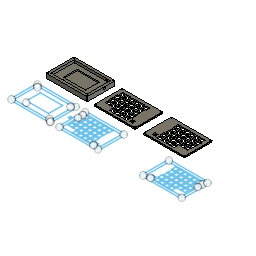
KEYBOARD_SPLIT (Autodesk Fusion 360 design; units mm, degrees)
part number: 2026-05-08-19-29-42-942
Autodesk Fusion 360 part; units mm, degrees
sketch "Sketch1" plane through (0, 0, 0) normal (0, 1, 0) x (1, 0, 0)
  line L0 (45, 19.9678) -> (192.4, 19.9678)
  line L1 (192.4, 19.9678) -> (192.4, -74.4322)
  line L2 (192.4, -74.4322) -> (45, -74.4322)
  line L3 (45, -74.4322) -> (45, 19.9678)
  line L4 (35, -84.4322) -> (35, 29.9678)
  line L5 (35, 29.9678) -> (202.4, 29.9678)
  line L6 (202.4, 29.9678) -> (202.4, -84.4322)
  line L7 (202.4, -84.4322) -> (35, -84.4322)
  line L8 (75, 2.7892) -> (165, 2.7892)
  line L9 (165, 2.7892) -> (165, -54.0461)
  line L10 (165, -54.0461) -> (75, -54.0461)
  line L11 (75, -54.0461) -> (75, 2.7892)
  line L12 (38, 27) -> (38, 23)
  line L13 (42, 23) -> (42, 27)
  line L14 (42, 27) -> (38, 27)
  line L15 (38, 23) -> (42, 23)
  line L16 (38, -78) -> (38, -82)
  line L17 (38, -82) -> (42, -82)
  line L18 (42, -82) -> (42, -78)
  line L19 (42, -78) -> (38, -78)
  line L20 (195.5084, -78) -> (195.5084, -82)
  line L21 (195.5084, -82) -> (199.5084, -82)
  line L22 (199.5084, -82) -> (199.5084, -78)
  line L23 (199.5084, -78) -> (195.5084, -78)
  line L24 (195.5084, 23.0262) -> (199.5084, 23.0262)
  line L25 (199.5084, 23.0262) -> (199.5084, 27.0262)
  line L26 (195.5084, 23.0262) -> (195.5084, 27.0262)
  line L27 (195.5084, 27.0262) -> (199.5084, 27.0262)
  point P0 (40, 25)
  point P1 (197.5, 25)
  point P2 (197.5, -80)
  point P3 (40, -80)
  point P4 (186.4, 13.9678)
  point P5 (186.4, -71.7)
  point P6 (80.7091, -61.1944)
  point P7 (49.5091, 16.0056)
  dimension "d1" = 147.4
  dimension "d2" = 94.4
  dimension "d3" = 147.4
  dimension "d6" = -10
  dimension "d24" = 4
  dimension "d25" = 4
  dimension "d26" = 4
  constraint horizontal L0
  constraint perpendicular L0 L1
  constraint perpendicular L1 L2
  constraint horizontal L8
  constraint vertical L9
  constraint horizontal L10
  constraint vertical L11
  constraint vertical L12
  constraint parallel L12 L13
  constraint perpendicular L13 L14
  constraint perpendicular L13 L15
  constraint perpendicular L15 L16
  constraint perpendicular L16 L17
  constraint perpendicular L17 L18
  constraint perpendicular L16 L19
  constraint vertical L20
  constraint perpendicular L20 L21
  constraint perpendicular L21 L22
  constraint perpendicular L20 L23
  constraint perpendicular L20 L24
  constraint perpendicular L24 L25
  constraint perpendicular L24 L26
  measures "d1" distance of L0.start L0.end
  measures "d2" distance of L0.end L1.end
  measures "d3" distance of L1.end L2.end
  measures "d24" distance of L24.start L24.end
  measures "d25" distance of L24.end L25.end
  measures "d26" distance of L24.start L26.end
extrude "Extrude1" add sketch "Sketch1" along normal blind 3 contours L0 L1 L2 L3 | L4 L5 L6 L7 | L8 L9 L10 L11 | L12 L13 L14 L15 | L16 L17 L18 L19 | L20 L21 L22 L23 | L24 L25 L26 L27 makes body 1
extrude "Extrude2" add sketch "Sketch1" along normal blind 8 separate body contours L0 L1 L2 L3 | L4 L5 L6 L7 | L12 L13 L14 L15 | L16 L17 L18 L19 | L20 L21 L22 L23 | L24 L25 L26 L27 makes body 2
extrude "Extrude3" add sketch "Sketch1" along normal blind 18 separate body contours L4 L5 L6 L7 | L12 L13 L14 L15 | L16 L17 L18 L19 | L20 L21 L22 L23 | L24 L25 L26 L27 makes body 3
combine "Combine1" operation add target body 1 tool bodies 2 3
hole "Hole1" at (49.5091, 0, -16.0056) at (80.7091, 0, 61.1944) at (186.4, 0, 71.7) at (186.4, 0, -13.9678) direction (0, 1, 0) diameter 2.4 end through all bodies 1
hole "Hole2" at (40, 0, -25) at (40, 0, 80) at (197.5, 0, -25) at (197.5, 0, 80) direction (0, 1, 0) diameter 2.4 end through all bodies 1
extrude "Extrude4" add sketch "Sketch1" along normal blind 3 separate body contours L12 L13 L14 L15 | L16 L17 L18 L19 | L20 L21 L22 L23 | L24 L25 L26 L27 makes body 4 at (196.8417, 0, 79.3333) makes body 5 at (39.3333, 0, 79.3333) makes body 6 at (196.8417, 0, -25.6929) makes body 7 at (39.3333, 0, -25.6667)
combine "Combine2" operation cut target body 1 tool bodies 4 5 6 7
sketch "Sketch2" plane through (0, 0, 0) normal (0, 1, 0) x (1, 0, 0)
  line L0 (220, 15) -> (229.1, 15)
  line L1 (229.1, 15) -> (229.1, -5)
  line L2 (229.1, -5) -> (220, -5)
  line L3 (220, -5) -> (220, 15)
  dimension "d29" = 9.1
  constraint horizontal L0
  constraint vertical L1
  constraint horizontal L2
  constraint vertical L3
  measures "d29" distance of L0.start L0.end
extrude "Extrude5" add sketch "Sketch2" along normal blind 3.4 separate body makes body 8
fillet "Fillet1" radius 0.5 4 edges at (229.1, 3.4, -5) (220, 3.4, -5) (229.1, 0, -5) (220, 0, -5) on bodies 8
move_body "Move1" bodies 8 to x (1, 0, 0) y (0, 1, 0) z (0, 0, 1) at (-48, 7.5, -20)
move_body "Move2" bodies 8 to x (1, 0, 0) y (0, 1, 0) z (0, 0, 1) at (0, 2, 0)
combine "Combine3" operation cut target body 1 tool bodies 8
fillet "Fillet2" radius 2 4 edges at (202.4, 9, -29.9678) (35, 9, -29.9678) (35, 9, 84.4322) (202.4, 9, 84.4322) on bodies 1
move_body "Move3" bodies 1 to x (1, 0, 0) y (0, 1, 0) z (0, 0, 1) at (0, 0, -150)
sketch "Sketch3" plane through (0, 0, 0) normal (0, 1, 0) x (1, 0, 0)
  line L0 (220, -20) -> (225, -20)
  line L1 (225, -20) -> (225, -28)
  line L2 (225, -28) -> (220, -28)
  line L3 (220, -28) -> (220, -20)
  dimension "d36" = 5
  dimension "d37" = 8
  constraint horizontal L0
  constraint vertical L1
  constraint horizontal L2
  constraint vertical L3
  measures "d36" distance of L0.start L0.end
  measures "d37" distance of L0.start L2.end
extrude "Extrude7" add sketch "Sketch3" along normal blind 20 separate body makes body 9
move_body "Move4" bodies 9 to x (0, 1, 0) y (-1, 0, 0) z (0, 0, 1) at (220, -220, 0)
move_body "Move5" bodies 9 to x (1, 0, 0) y (0, 1, 0) z (0, 0, 1) at (15, 10, -150)
move_body "Move6" bodies 9 to x (1, 0, 0) y (0, 1, 0) z (0, 0, 1) at (-27, -2, -12)
move_body "Move7" bodies 9 to x (1, 0, 0) y (0, 1, 0) z (0, 0, 1) at (0, 1, 0)
combine "Combine4" operation cut target body 1 tool bodies 9
sketch "Sketch4Sketch4" plane through (0, 0, 0) normal (0, 1, 0) x (1, 0, 0)
  line L0 (240, 20) -> (387.4, 20)
  line L1 (240, 20) -> (240, -74.4)
  line L2 (387.4, 20) -> (387.4, -74.4)
  line L3 (240, -74.4) -> (387.4, -74.4)
  line L4 (397.4, 30) -> (397.4, -84.4)
  line L5 (230, -84.4) -> (397.4, -84.4)
  line L6 (230, 30) -> (230, -84.4)
  line L7 (230, 30) -> (397.4, 30)
  line L8 (240, 20) -> (240, 9.6)
  line L9 (246.65, 9.6) -> (246.65, 16.65)
  line L10 (246.65, 16.65) -> (260.75, 16.65)
  line L11 (260.75, 16.65) -> (260.75, 2.55)
  line L12 (260.75, 2.55) -> (246.65, 2.55)
  line L13 (246.65, 2.55) -> (246.65, 9.6)
  line L14 (265.7, 16.65) -> (279.8, 16.65)
  line L15 (279.8, 16.65) -> (279.8, 2.55)
  line L16 (279.8, 2.55) -> (265.7, 2.55)
  line L17 (265.7, 2.55) -> (265.7, 16.65)
  line L18 (284.7517, 16.65) -> (298.8517, 16.65)
  line L19 (298.8517, 16.65) -> (298.8517, 2.55)
  line L20 (298.8517, 2.55) -> (284.7517, 2.55)
  line L21 (284.7517, 2.55) -> (284.7517, 16.65)
  line L22 (303.8299, 16.65) -> (317.9299, 16.65)
  line L23 (317.9299, 16.65) -> (317.9299, 2.65)
  line L24 (317.9299, 2.65) -> (303.8299, 2.65)
  line L25 (303.8299, 2.65) -> (303.8299, 16.65)
  line L26 (322.8799, 2.65) -> (322.8799, 16.65)
  line L27 (322.8799, 16.65) -> (336.9799, 16.65)
  line L28 (336.9799, 2.65) -> (322.8799, 2.65)
  line L29 (336.9799, 16.65) -> (336.9799, 2.65)
  line L30 (341.9299, 2.65) -> (341.9299, 16.65)
  line L31 (341.9299, 16.65) -> (356.0299, 16.65)
  line L32 (356.0299, 2.65) -> (341.9299, 2.65)
  line L33 (356.0299, 16.65) -> (356.0299, 2.65)
  line L34 (240, 20) -> (240, -9.43)
  line L35 (244.12, -9.43) -> (244.12, -2.38)
  line L36 (244.12, -2.38) -> (258.22, -2.38)
  line L37 (258.22, -2.38) -> (258.22, -16.48)
  line L38 (258.22, -16.48) -> (244.12, -16.48)
  line L39 (244.12, -16.48) -> (244.12, -9.43)
  line L40 (263.0302, -2.38) -> (277.1302, -2.38)
  line L41 (277.1302, -2.38) -> (277.1302, -16.48)
  line L42 (277.1302, -16.48) -> (263.0302, -16.48)
  line L43 (263.0302, -16.48) -> (263.0302, -2.38)
  line L44 (282.0802, -16.48) -> (282.0802, -2.38)
  line L45 (282.0802, -2.38) -> (296.1802, -2.38)
  line L46 (296.1802, -2.38) -> (296.1802, -16.48)
  line L47 (296.1802, -16.48) -> (282.0802, -16.48)
  line L48 (301.1302, -16.48) -> (301.1302, -2.38)
  line L49 (315.2302, -16.48) -> (301.1302, -16.48)
  line L50 (315.2302, -2.38) -> (315.2302, -16.48)
  line L51 (301.1302, -2.38) -> (315.2302, -2.38)
  line L52 (320.1802, -16.48) -> (320.1802, -2.38)
  line L53 (320.1802, -2.38) -> (334.2802, -2.38)
  line L54 (334.2802, -16.48) -> (320.1802, -16.48)
  line L55 (334.2802, -2.38) -> (334.2802, -16.48)
  line L56 (339.2302, -16.48) -> (339.2302, -2.38)
  line L57 (353.3302, -16.48) -> (339.2302, -16.48)
  line L58 (353.3302, -2.38) -> (353.3302, -16.48)
  line L59 (339.2302, -2.38) -> (353.3302, -2.38)
  line L60 (244.12, -21.43) -> (258.22, -21.43)
  line L61 (244.12, -28.48) -> (244.12, -21.43)
  line L62 (244.12, -35.53) -> (244.12, -28.48)
  line L63 (258.22, -21.43) -> (258.22, -35.53)
  line L64 (277.1302, -21.43) -> (277.1302, -35.53)
  line L65 (258.22, -35.53) -> (244.12, -35.53)
  line L66 (263.0302, -35.53) -> (263.0302, -21.43)
  line L67 (263.0302, -21.43) -> (277.1302, -21.43)
  line L68 (282.0802, -35.53) -> (282.0802, -21.43)
  line L69 (277.1302, -35.53) -> (263.0302, -35.53)
  line L70 (339.2302, -35.53) -> (339.2302, -21.43)
  line L71 (301.1302, -21.43) -> (315.2302, -21.43)
  line L72 (315.2302, -21.43) -> (315.2302, -35.53)
  line L73 (353.3302, -21.43) -> (353.3302, -35.53)
  line L74 (315.2302, -35.53) -> (301.1302, -35.53)
  line L75 (339.2302, -21.43) -> (353.3302, -21.43)
  line L76 (320.1802, -35.53) -> (320.1802, -21.43)
  line L77 (334.2802, -21.43) -> (334.2802, -35.53)
  line L78 (334.2802, -35.53) -> (320.1802, -35.53)
  line L79 (353.3302, -35.53) -> (339.2302, -35.53)
  line L80 (320.1802, -21.43) -> (334.2802, -21.43)
  line L81 (301.1302, -35.53) -> (301.1302, -21.43)
  line L82 (296.1802, -21.43) -> (296.1802, -35.53)
  line L83 (296.1802, -35.53) -> (282.0802, -35.53)
  line L84 (282.0802, -21.43) -> (296.1802, -21.43)
  line L85 (246.65, -54.6) -> (246.65, -47.55)
  line L86 (265.7, -54.6) -> (265.7, -40.5)
  line L87 (265.7, -40.5) -> (279.8, -40.5)
  line L88 (260.75, -40.5) -> (260.75, -54.6)
  line L89 (246.65, -40.5) -> (260.75, -40.5)
  line L90 (260.75, -54.6) -> (246.65, -54.6)
  line L91 (279.8, -54.6) -> (265.7, -54.6)
  line L92 (284.7517, -54.6) -> (284.7517, -40.5)
  line L93 (279.8, -40.5) -> (279.8, -54.6)
  line L94 (246.65, -47.55) -> (246.65, -40.5)
  line L95 (284.7517, -40.5) -> (298.8517, -40.5)
  line L96 (298.8517, -54.6) -> (284.7517, -54.6)
  line L97 (356.0299, -54.5) -> (341.9299, -54.5)
  line L98 (322.8799, -40.5) -> (336.9799, -40.5)
  line L99 (336.9799, -54.5) -> (322.8799, -54.5)
  line L100 (336.9799, -40.5) -> (336.9799, -54.5)
  line L101 (341.9299, -40.5) -> (356.0299, -40.5)
  line L102 (322.8799, -54.5) -> (322.8799, -40.5)
  line L103 (303.8299, -40.5) -> (317.9299, -40.5)
  line L104 (356.0299, -40.5) -> (356.0299, -54.5)
  line L105 (317.9299, -40.5) -> (317.9299, -54.5)
  line L106 (317.9299, -54.5) -> (303.8299, -54.5)
  line L107 (303.8299, -54.5) -> (303.8299, -40.5)
  line L108 (298.8517, -40.5) -> (298.8517, -54.6)
  line L109 (341.9299, -54.5) -> (341.9299, -40.5)
  line L110 (334.2802, -73.63) -> (320.1802, -73.63)
  line L111 (334.2802, -59.53) -> (334.2802, -73.63)
  line L112 (296.1802, -73.63) -> (282.0802, -73.63)
  line L113 (315.2302, -73.63) -> (301.1302, -73.63)
  line L114 (315.2302, -59.53) -> (315.2302, -73.63)
  line L115 (282.0802, -59.53) -> (296.1802, -59.53)
  line L116 (282.0802, -73.63) -> (282.0802, -59.53)
  line L117 (296.1802, -59.53) -> (296.1802, -73.63)
  line L118 (301.1302, -59.53) -> (315.2302, -59.53)
  line L119 (320.1802, -73.63) -> (320.1802, -59.53)
  line L120 (339.2302, -73.63) -> (339.2302, -59.53)
  line L121 (353.3302, -59.53) -> (353.3302, -73.63)
  line L122 (353.3302, -73.63) -> (339.2302, -73.63)
  line L123 (339.2302, -59.53) -> (353.3302, -59.53)
  line L124 (301.1302, -73.63) -> (301.1302, -59.53)
  line L125 (320.1802, -59.53) -> (334.2802, -59.53)
  line L126 (387.4, -74.4) -> (368.2, -74.4)
  line L127 (374.3932, -71.2) -> (361.9932, -71.2)
  line L128 (361.9932, -71.2) -> (361.9932, -59.4)
  line L129 (361.9932, -59.4) -> (374.3932, -59.4)
  line L130 (374.3932, -59.4) -> (374.3932, -71.2)
  line L131 (594.3932, -71.2) -> (606.7932, -71.2)
  line L132 (691.6561, -16.48) -> (705.7561, -16.48)
  line L133 (722.1363, -40.5) -> (708.0363, -40.5)
  line L134 (705.7561, -35.53) -> (705.7561, -21.43)
  line L135 (691.6561, -35.53) -> (705.7561, -35.53)
  line L136 (724.6663, -9.43) -> (724.6663, -2.38)
  line L137 (724.6663, -35.53) -> (724.6663, -28.48)
  line L138 (722.1363, 9.6) -> (722.1363, 16.65)
  line L139 (669.9346, -54.6) -> (684.0346, -54.6)
  line L140 (705.7561, -21.43) -> (691.6561, -21.43)
  line L141 (722.1363, 2.55) -> (722.1363, 9.6)
  line L142 (688.9863, -40.5) -> (688.9863, -54.6)
  line L143 (686.7061, -21.43) -> (672.6061, -21.43)
  line L144 (703.0863, -40.5) -> (688.9863, -40.5)
  line L145 (722.1363, 16.65) -> (708.0363, 16.65)
  line L146 (728.7863, 20) -> (728.7863, -9.43)
  line L147 (703.0863, -54.6) -> (703.0863, -40.5)
  line L148 (722.1363, -47.55) -> (722.1363, -40.5)
  line L149 (703.0863, 2.55) -> (703.0863, 16.65)
  line L150 (686.7061, -35.53) -> (686.7061, -21.43)
  line L151 (722.1363, -54.6) -> (722.1363, -47.55)
  line L152 (684.0346, 2.55) -> (684.0346, 16.65)
  line L153 (710.5663, -21.43) -> (710.5663, -35.53)
  line L154 (710.5663, -16.48) -> (724.6663, -16.48)
  line L155 (710.5663, -35.53) -> (724.6663, -35.53)
  line L156 (688.9863, 2.55) -> (703.0863, 2.55)
  line L157 (724.6663, -2.38) -> (710.5663, -2.38)
  line L158 (708.0363, -54.6) -> (722.1363, -54.6)
  line L159 (688.9863, 16.65) -> (688.9863, 2.55)
  line L160 (703.0863, 16.65) -> (688.9863, 16.65)
  line L161 (708.0363, 2.55) -> (722.1363, 2.55)
  line L162 (724.6663, -28.48) -> (724.6663, -21.43)
  line L163 (581.3863, 20) -> (581.3863, -74.4)
  line L164 (653.5561, -2.38) -> (653.5561, -16.48)
  line L165 (571.3863, 30) -> (571.3863, -84.4)
  line L166 (686.7061, -73.63) -> (686.7061, -59.53)
  line L167 (667.6561, -16.48) -> (667.6561, -2.38)
  line L168 (724.6663, -21.43) -> (710.5663, -21.43)
  line L169 (648.6061, -2.38) -> (634.5061, -2.38)
  line L170 (631.8064, 2.65) -> (645.9064, 2.65)
  line L171 (669.9346, 16.65) -> (669.9346, 2.55)
  line L172 (629.5561, -16.48) -> (629.5561, -2.38)
  line L173 (615.4561, -2.38) -> (615.4561, -16.48)
  line L174 (645.9064, 2.65) -> (645.9064, 16.65)
  line L175 (667.6561, -2.38) -> (653.5561, -2.38)
  line L176 (664.9564, 16.65) -> (650.8564, 16.65)
  line L177 (684.0346, -54.6) -> (684.0346, -40.5)
  line L178 (708.0363, -40.5) -> (708.0363, -54.6)
  line L179 (648.6061, -16.48) -> (648.6061, -2.38)
  line L180 (672.6061, -2.38) -> (672.6061, -16.48)
  line L181 (634.5061, -2.38) -> (634.5061, -16.48)
  line L182 (650.8564, 2.65) -> (664.9564, 2.65)
  line L183 (688.9863, -54.6) -> (703.0863, -54.6)
  line L184 (645.9064, 16.65) -> (631.8064, 16.65)
  line L185 (691.6561, -21.43) -> (691.6561, -35.53)
  line L186 (667.6561, -21.43) -> (653.5561, -21.43)
  line L187 (664.9564, -40.5) -> (650.8564, -40.5)
  line L188 (653.5561, -59.53) -> (653.5561, -73.63)
  line L189 (612.7564, 16.65) -> (612.7564, 2.65)
  line L190 (631.8064, -54.5) -> (645.9064, -54.5)
  line L191 (612.7564, 2.65) -> (626.8564, 2.65)
  line L192 (626.8564, 16.65) -> (612.7564, 16.65)
  line L193 (631.8064, 16.65) -> (631.8064, 2.65)
  line L194 (664.9564, 2.65) -> (664.9564, 16.65)
  line L195 (653.5561, -73.63) -> (667.6561, -73.63)
  line L196 (650.8564, -54.5) -> (664.9564, -54.5)
  line L197 (645.9064, -40.5) -> (631.8064, -40.5)
  line L198 (650.8564, -40.5) -> (650.8564, -54.5)
  line L199 (648.6061, -59.53) -> (634.5061, -59.53)
  line L200 (667.6561, -73.63) -> (667.6561, -59.53)
  line L201 (667.6561, -59.53) -> (653.5561, -59.53)
  line L202 (626.8564, 2.65) -> (626.8564, 16.65)
  line L203 (629.5561, -2.38) -> (615.4561, -2.38)
  line L204 (634.5061, -73.63) -> (648.6061, -73.63)
  line L205 (650.8564, 16.65) -> (650.8564, 2.65)
  line L206 (645.9064, -54.5) -> (645.9064, -40.5)
  line L207 (648.6061, -35.53) -> (648.6061, -21.43)
  line L208 (669.9346, -40.5) -> (669.9346, -54.6)
  line L209 (634.5061, -16.48) -> (648.6061, -16.48)
  line L210 (648.6061, -21.43) -> (634.5061, -21.43)
  line L211 (664.9564, -54.5) -> (664.9564, -40.5)
  line L212 (653.5561, -16.48) -> (667.6561, -16.48)
  line L213 (672.6061, -59.53) -> (672.6061, -73.63)
  line L214 (653.5561, -35.53) -> (667.6561, -35.53)
  line L215 (634.5061, -35.53) -> (648.6061, -35.53)
  line L216 (615.4561, -21.43) -> (615.4561, -35.53)
  line L217 (615.4561, -16.48) -> (629.5561, -16.48)
  line L218 (606.7932, -71.2) -> (606.7932, -59.4)
  line L219 (612.7564, -40.5) -> (612.7564, -54.5)
  line L220 (672.6061, -21.43) -> (672.6061, -35.53)
  line L221 (634.5061, -21.43) -> (634.5061, -35.53)
  line L222 (667.6561, -35.53) -> (667.6561, -21.43)
  line L223 (631.8064, -40.5) -> (631.8064, -54.5)
  line L224 (634.5061, -59.53) -> (634.5061, -73.63)
  line L225 (653.5561, -21.43) -> (653.5561, -35.53)
  line L226 (626.8564, -40.5) -> (612.7564, -40.5)
  line L227 (615.4561, -73.63) -> (629.5561, -73.63)
  line L228 (648.6061, -73.63) -> (648.6061, -59.53)
  line L229 (626.8564, -54.5) -> (626.8564, -40.5)
  line L230 (612.7564, -54.5) -> (626.8564, -54.5)
  line L231 (594.3932, -59.4) -> (594.3932, -71.2)
  line L232 (615.4561, -59.53) -> (615.4561, -73.63)
  line L233 (629.5561, -21.43) -> (615.4561, -21.43)
  line L234 (581.3863, -74.4) -> (600.5863, -74.4)
  line L235 (629.5561, -35.53) -> (629.5561, -21.43)
  line L236 (629.5561, -59.53) -> (615.4561, -59.53)
  line L237 (606.7932, -59.4) -> (594.3932, -59.4)
  line L238 (615.4561, -35.53) -> (629.5561, -35.53)
  line L239 (629.5561, -73.63) -> (629.5561, -59.53)
  line L240 (738.7863, 30) -> (571.3863, 30)
  line L241 (672.6061, -16.48) -> (686.7061, -16.48)
  line L242 (686.7061, -2.38) -> (672.6061, -2.38)
  line L243 (686.7061, -59.53) -> (672.6061, -59.53)
  line L244 (684.0346, 16.65) -> (669.9346, 16.65)
  line L245 (738.7863, -84.4) -> (571.3863, -84.4)
  line L246 (691.6561, -2.38) -> (691.6561, -16.48)
  line L247 (710.5663, -2.38) -> (710.5663, -16.48)
  line L248 (708.0363, 16.65) -> (708.0363, 2.55)
  line L249 (705.7561, -16.48) -> (705.7561, -2.38)
  line L250 (728.7863, 20) -> (728.7863, 9.6)
  line L251 (672.6061, -73.63) -> (686.7061, -73.63)
  line L252 (684.0346, -40.5) -> (669.9346, -40.5)
  line L253 (728.7863, 20) -> (728.7863, -74.4)
  line L254 (672.6061, -35.53) -> (686.7061, -35.53)
  line L255 (724.6663, -16.48) -> (724.6663, -9.43)
  line L256 (738.7863, 30) -> (738.7863, -84.4)
  line L257 (669.9346, 2.55) -> (684.0346, 2.55)
  line L258 (728.7863, -74.4) -> (581.3863, -74.4)
  line L259 (705.7561, -2.38) -> (691.6561, -2.38)
  line L260 (728.7863, 20) -> (581.3863, 20)
  line L261 (686.7061, -16.48) -> (686.7061, -2.38)
  point P0 (197.5, -80)
  point P1 (235, -80)
  point P2 (235, 25)
  point P3 (392.4, 25)
  point P4 (392.4, -80)
  point P5 (733.7863, -80)
  point P6 (733.7863, 25)
  point P7 (576.3863, 25)
  point P8 (576.3863, -80)
  dimension "d42" = 147.4
  dimension "d44" = 94.4
  dimension "d45" = 10
  dimension "d46" = 10.4
  dimension "d50" = 7.05
  dimension "d51" = 14.1
  dimension "d52" = 14.1
  dimension "d53" = 14.1
  dimension "d55" = 14.1
  dimension "d56" = 14.1
  dimension "d59" = 14.1
  dimension "d60" = 14.1
  dimension "d63" = 14
  dimension "d64" = 14.1
  dimension "d66" = 14
  dimension "d67" = 14.1
  dimension "d69" = 14
  dimension "d70" = 14.1
  dimension "d71" = 29.43
  dimension "d74" = 7.05
  dimension "d75" = 14.1
  dimension "d76" = 14.1
  dimension "d77" = 14.1
  dimension "d80" = 14.1
  dimension "d81" = 14.1
  dimension "d83" = 14.1
  dimension "d84" = 14.1
  dimension "d85" = 14.1
  dimension "d86" = 14.1
  dimension "d87" = 14.1
  dimension "d88" = 14.1
  dimension "d89" = 14.1
  dimension "d90" = 14.1
  dimension "d92" = 7.05
  dimension "d93" = 14.1
  dimension "d94" = 14.1
  dimension "d95" = 14.1
  dimension "d98" = 14.1
  dimension "d99" = 14.1
  dimension "d101" = 14.1
  dimension "d102" = 14.1
  dimension "d103" = 14.1
  dimension "d104" = 14.1
  dimension "d105" = 14.1
  dimension "d106" = 14.1
  dimension "d107" = 14.1
  dimension "d108" = 14.1
  dimension "d111" = 7.05
  dimension "d112" = 14.1
  dimension "d113" = 14.1
  dimension "d114" = 14.1
  dimension "d116" = 14.1
  dimension "d117" = 14.1
  dimension "d120" = 14.1
  dimension "d121" = 14.1
  dimension "d124" = 14
  dimension "d125" = 14.1
  dimension "d127" = 14
  dimension "d128" = 14.1
  dimension "d130" = 14
  dimension "d131" = 14.1
  dimension "d133" = 14.1
  dimension "d134" = 14.1
  dimension "d135" = 14.1
  dimension "d136" = 14.1
  dimension "d137" = 14.1
  dimension "d138" = 14.1
  dimension "d139" = 14.1
  dimension "d140" = 14.1
  dimension "d141" = 19.2
  dimension "d145" = 11.8
  dimension "d146" = 12.4
  dimension "d155" = 10
  dimension "d156" = 147.4
  dimension "d157" = 94.4
  dimension "d158" = 10.4
  dimension "d159" = 7.05
  dimension "d160" = 14.1
  dimension "d161" = 14.1
  dimension "d162" = 14.1
  dimension "d163" = 14.1
  dimension "d164" = 14.1
  dimension "d165" = 14.1
  dimension "d166" = 14.1
  dimension "d167" = 14
  dimension "d168" = 14.1
  dimension "d169" = 14
  dimension "d170" = 14.1
  dimension "d171" = 14
  dimension "d172" = 14.1
  dimension "d173" = 29.43
  dimension "d174" = 7.05
  dimension "d175" = 14.1
  dimension "d176" = 14.1
  dimension "d177" = 14.1
  dimension "d178" = 14.1
  dimension "d179" = 14.1
  dimension "d180" = 14.1
  dimension "d181" = 14.1
  dimension "d182" = 14.1
  dimension "d183" = 14.1
  dimension "d184" = 14.1
  dimension "d185" = 14.1
  dimension "d186" = 14.1
  dimension "d187" = 14.1
  dimension "d188" = 7.05
  dimension "d189" = 14.1
  dimension "d190" = 14.1
  dimension "d191" = 14.1
  dimension "d192" = 14.1
  dimension "d193" = 14.1
  dimension "d194" = 14.1
  dimension "d195" = 14.1
  dimension "d196" = 14.1
  dimension "d197" = 14.1
  dimension "d198" = 14.1
  dimension "d199" = 14.1
  dimension "d200" = 14.1
  dimension "d201" = 14.1
  dimension "d202" = 7.05
  dimension "d203" = 14.1
  dimension "d204" = 14.1
  dimension "d205" = 14.1
  dimension "d206" = 14.1
  dimension "d207" = 14.1
  dimension "d208" = 14.1
  dimension "d209" = 14.1
  dimension "d210" = 14
  dimension "d211" = 14.1
  dimension "d212" = 14
  dimension "d213" = 14.1
  dimension "d214" = 14
  dimension "d215" = 14.1
  dimension "d216" = 14.1
  dimension "d217" = 14.1
  dimension "d218" = 14.1
  dimension "d219" = 14.1
  dimension "d220" = 14.1
  dimension "d221" = 14.1
  dimension "d222" = 14.1
  dimension "d223" = 14.1
  dimension "d224" = 19.2
  dimension "d225" = 11.8
  dimension "d226" = 12.4
  constraint horizontal L0
  constraint perpendicular L0 L1
  constraint perpendicular L0 L2
  constraint perpendicular L2 L3
  constraint perpendicular L0 L8
  constraint perpendicular L9 L10
  constraint perpendicular L10 L11
  constraint perpendicular L11 L12
  constraint horizontal L14
  constraint vertical L15
  constraint horizontal L16
  constraint vertical L17
  constraint horizontal L18
  constraint vertical L19
  constraint horizontal L20
  constraint vertical L21
  constraint horizontal L22
  constraint vertical L23
  constraint horizontal L24
  constraint vertical L25
  constraint horizontal L27
  constraint vertical L29
  constraint horizontal L28
  constraint vertical L26
  constraint horizontal L31
  constraint vertical L33
  constraint horizontal L32
  constraint vertical L30
  constraint perpendicular L35 L36
  constraint perpendicular L36 L37
  constraint perpendicular L37 L38
  constraint horizontal L40
  constraint vertical L41
  constraint horizontal L42
  constraint vertical L43
  constraint horizontal L45
  constraint vertical L46
  constraint horizontal L47
  constraint vertical L44
  constraint horizontal L51
  constraint vertical L50
  constraint horizontal L49
  constraint vertical L48
  constraint horizontal L53
  constraint vertical L55
  constraint horizontal L54
  constraint vertical L52
  constraint horizontal L59
  constraint vertical L58
  constraint horizontal L57
  constraint vertical L56
  constraint perpendicular L60 L61
  constraint perpendicular L60 L63
  constraint perpendicular L63 L65
  constraint horizontal L67
  constraint vertical L64
  constraint horizontal L69
  constraint vertical L66
  constraint horizontal L84
  constraint vertical L82
  constraint horizontal L83
  constraint vertical L68
  constraint horizontal L71
  constraint vertical L72
  constraint horizontal L74
  constraint vertical L81
  constraint horizontal L80
  constraint vertical L77
  constraint horizontal L78
  constraint vertical L76
  constraint horizontal L75
  constraint vertical L73
  constraint horizontal L79
  constraint vertical L70
  constraint perpendicular L89 L94
  constraint perpendicular L88 L89
  constraint perpendicular L88 L90
  constraint horizontal L87
  constraint vertical L93
  constraint horizontal L91
  constraint vertical L86
  constraint horizontal L95
  constraint vertical L108
  constraint horizontal L96
  constraint vertical L92
  constraint horizontal L103
  constraint vertical L105
  constraint horizontal L106
  constraint vertical L107
  constraint horizontal L98
  constraint vertical L100
  constraint horizontal L99
  constraint vertical L102
  constraint horizontal L101
  constraint vertical L104
  constraint horizontal L97
  constraint vertical L109
  constraint horizontal L115
  constraint vertical L117
  constraint horizontal L112
  constraint vertical L116
  constraint horizontal L118
  constraint vertical L114
  constraint horizontal L113
  constraint vertical L124
  constraint horizontal L125
  constraint vertical L111
  constraint horizontal L110
  constraint vertical L119
  constraint horizontal L123
  constraint vertical L121
  constraint horizontal L122
  constraint vertical L120
  constraint perpendicular L2 L126
  constraint horizontal L127
  constraint vertical L128
  constraint horizontal L129
  constraint vertical L130
  constraint perpendicular L253 L260
  constraint perpendicular L163 L260
  constraint perpendicular L163 L258
  constraint perpendicular L250 L260
  constraint perpendicular L138 L145
  constraint perpendicular L145 L248
  constraint perpendicular L161 L248
  constraint perpendicular L136 L157
  constraint perpendicular L157 L247
  constraint perpendicular L154 L247
  constraint perpendicular L162 L168
  constraint perpendicular L153 L168
  constraint perpendicular L153 L155
  constraint perpendicular L133 L148
  constraint perpendicular L133 L178
  constraint perpendicular L158 L178
  constraint perpendicular L163 L234
  measures "d42" distance of L0.start L0.end
  measures "d44" distance of L0.end L2.end
  measures "d46" distance of L0.start L8.end
  measures "d50" distance of L9.start L9.end
  measures "d51" distance of L9.end L10.end
  measures "d52" distance of L10.end L11.end
  measures "d53" distance of L11.end L12.end
  measures "d55" distance of L14.start L16.end
  measures "d56" distance of L14.start L14.end
  measures "d59" distance of L18.start L20.end
  measures "d60" distance of L18.start L18.end
  measures "d63" distance of L22.start L24.end
  measures "d64" distance of L22.start L22.end
  measures "d66" distance of L26.start L26.end
  measures "d67" distance of L27.end L26.end
  measures "d69" distance of L30.start L30.end
  measures "d70" distance of L31.end L30.end
  measures "d71" distance of L0.start L34.end
  measures "d74" distance of L35.start L35.end
  measures "d75" distance of L35.end L36.end
  measures "d76" distance of L36.end L37.end
  measures "d77" distance of L37.end L38.end
  measures "d80" distance of L40.start L42.end
  measures "d81" distance of L40.start L40.end
  measures "d83" distance of L44.end L44.start
  measures "d84" distance of L44.end L45.end
  measures "d85" distance of L48.end L48.start
  measures "d86" distance of L48.end L50.start
  measures "d87" distance of L52.start L52.end
  measures "d88" distance of L53.end L52.end
  measures "d89" distance of L56.end L56.start
  measures "d90" distance of L58.start L56.end
  measures "d92" distance of L60.start L61.start
  measures "d93" distance of L60.start L60.end
  measures "d94" distance of L63.end L60.end
  measures "d95" distance of L63.end L62.start
  measures "d98" distance of L66.end L66.start
  measures "d99" distance of L66.end L64.start
  measures "d101" distance of L68.end L68.start
  measures "d102" distance of L68.end L82.start
  measures "d103" distance of L74.end L71.start
  measures "d104" distance of L71.end L71.start
  measures "d105" distance of L76.end L76.start
  measures "d106" distance of L77.start L76.end
  measures "d107" distance of L70.end L70.start
  measures "d108" distance of L73.start L70.end
  measures "d111" distance of L85.end L89.start
  measures "d112" distance of L88.start L89.start
  measures "d113" distance of L88.start L88.end
  measures "d114" distance of L85.start L88.end
  measures "d116" distance of L86.start L86.end
  measures "d117" distance of L87.end L86.end
  measures "d120" distance of L92.end L92.start
  measures "d121" distance of L92.end L95.end
  measures "d124" distance of L106.end L103.start
  measures "d125" distance of L103.end L103.start
  measures "d127" distance of L98.start L99.end
  measures "d128" distance of L98.start L98.end
  measures "d130" distance of L101.start L97.end
  measures "d131" distance of L101.start L101.end
  measures "d133" distance of L115.start L112.end
  measures "d134" distance of L115.start L115.end
  measures "d135" distance of L118.start L113.end
  measures "d136" distance of L114.start L118.start
  measures "d137" distance of L119.end L110.end
  measures "d138" distance of L119.end L111.start
  measures "d139" distance of L120.end L120.start
  measures "d140" distance of L120.end L121.start
  measures "d141" distance of L2.end L126.end
  measures "d145" distance of L127.start L129.end
  measures "d146" distance of L128.end L129.end
  measures "d156" distance of L146.start L163.start
  measures "d157" distance of L163.start L163.end
  measures "d158" distance of L146.start L250.end
  measures "d159" distance of L138.start L138.end
  measures "d160" distance of L145.end L138.end
  measures "d161" distance of L145.end L161.start
  measures "d162" distance of L141.start L161.start
  measures "d163" distance of L149.start L149.end
  measures "d164" distance of L159.start L149.end
  measures "d165" distance of L152.end L152.start
  measures "d166" distance of L152.end L171.start
  measures "d167" distance of L182.end L176.start
  measures "d168" distance of L176.end L176.start
  measures "d169" distance of L174.end L170.end
  measures "d170" distance of L174.end L184.end
  measures "d171" distance of L192.start L191.end
  measures "d172" distance of L192.start L189.start
  measures "d173" distance of L146.start L146.end
  measures "d174" distance of L136.end L136.start
  measures "d175" distance of L136.end L157.end
  measures "d176" distance of L154.start L157.end
  measures "d177" distance of L154.start L154.end
  measures "d178" distance of L249.end L132.end
  measures "d179" distance of L249.end L246.start
  measures "d180" distance of L242.start L241.end
  measures "d181" distance of L242.start L180.start
  measures "d182" distance of L167.start L167.end
  measures "d183" distance of L164.start L167.end
  measures "d184" distance of L169.start L179.start
  measures "d185" distance of L169.end L169.start
  measures "d186" distance of L172.end L172.start
  measures "d187" distance of L173.start L172.end
  measures "d188" distance of L137.end L162.end
  measures "d189" distance of L162.end L153.start
  measures "d190" distance of L153.end L153.start
  measures "d191" distance of L153.end L137.start
  measures "d192" distance of L134.end L134.start
  measures "d193" distance of L134.end L140.end
  measures "d194" distance of L143.start L150.start
  measures "d195" distance of L143.start L143.end
  measures "d196" distance of L186.start L214.end
  measures "d197" distance of L186.end L186.start
  measures "d198" distance of L207.end L207.start
  measures "d199" distance of L207.end L210.end
  measures "d200" distance of L233.start L235.start
  measures "d201" distance of L233.start L216.start
  measures "d202" distance of L133.start L148.start
  measures "d203" distance of L133.start L133.end
  measures "d204" distance of L133.end L158.start
  measures "d205" distance of L151.start L158.start
  measures "d206" distance of L147.start L144.start
  measures "d207" distance of L142.start L144.start
  measures "d208" distance of L139.end L177.end
  measures "d209" distance of L177.end L208.start
  measures "d210" distance of L196.end L187.start
  measures "d211" distance of L187.end L187.start
  measures "d212" distance of L190.end L197.start
  measures "d213" distance of L197.start L197.end
  measures "d214" distance of L226.start L229.start
  measures "d215" distance of L219.start L226.start
  measures "d216" distance of L166.end L166.start
  measures "d217" distance of L166.end L213.start
  measures "d218" distance of L195.end L200.end
  measures "d219" distance of L188.start L200.end
  measures "d220" distance of L199.start L204.end
  measures "d221" distance of L199.start L199.end
  measures "d222" distance of L227.end L236.start
  measures "d223" distance of L232.start L236.start
  measures "d224" distance of L163.end L234.end
  measures "d225" distance of L231.start L131.start
  measures "d226" distance of L231.start L218.end
extrude "Extrude8" add sketch "Sketch4Sketch4" along normal blind 5 separate body contours L0 L1 L2 L3 L8 L34 L126 | L4 L5 L6 L7 makes body 10
hole "Hole3" at (392.4, 0, -25) at (392.4, 0, 80) at (235, 0, 80) at (235, 0, -25) direction (0, 1, 0) diameter 2.4 end through all bodies 10
fillet "Fillet3" radius 2 4 edges at (397.4, 2.5, 84.4) (230, 2.5, -30) (397.4, 2.5, -30) (230, 2.5, 84.4) on bodies 10
fillet "Fillet4" radius 1 8 edges at (396.8142, 5, 83.8142) (397.4, 5, 27.2) (396.8142, 5, -29.4142) (313.7, 5, -30) (230.5858, 5, -29.4142) (230, 5, 27.2) (230.5858, 5, 83.8142) (313.7, 5, 84.4) on bodies 10
move_body "Move8" bodies 10 to x (1, 0, 0) y (0, 1, 0) z (0, 0, 1) at (0, 0, -150)
extrude "Extrude9" add sketch "Sketch4Sketch4" along normal blind 5 separate body contours L146 L163 L234 L250 L253 L258 L260 | L165 L240 L245 L256 makes body 11
move_body "Move9" bodies 11 to x (1, 0, 0) y (0, 1, 0) z (0, 0, 1) at (0, -5, 0)
hole "Hole4" at (576.3863, 0, -25) at (576.3863, 0, 80) at (733.7863, 0, 80) at (733.7863, 0, -25) direction (0, -1, 0) diameter 2.4 end through all countersink diameter 2.7 countersink angle 90 bodies 11
fillet "Fillet5" radius 2 4 edges at (738.7863, -2.5, 84.4) (571.3863, -2.5, 84.4) (571.3863, -2.5, -30) (738.7863, -2.5, -30) on bodies 11
fillet "Fillet6" radius 1 8 edges at (738.2005, 0, -29.4142) (655.0863, 0, -30) (571.9721, 0, -29.4142) (571.3863, 0, 27.2) (571.9721, 0, 83.8142) (655.0863, 0, 84.4) (738.2005, 0, 83.8142) (738.7863, 0, 27.2) on bodies 11
move_body "Move10" bodies 11 to x (1, 0, 0) y (0, 1, 0) z (0, 0, 1) at (0, 5, 0)
move_body "Move11" bodies 11 to x (1, 0, 0) y (0, 1, 0) z (0, 0, 1) at (-140, 0, -150)
